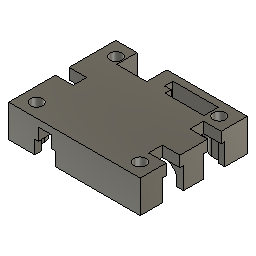
cover servo module (Autodesk Fusion 360 design; units mm, degrees)
Autodesk Fusion 360 part; units mm, degrees
note: some values were not read from the file. Set by a fixed rule: which sketch regions a step uses.
sketch "Skizze1" plane through (0, 0, 0) normal (0, 0, 1) x (1, 0, 0)
  line L0 (24.25, -19.75) -> (-24.25, -19.75)
  line L1 (-24.25, -19.75) -> (-24.25, 19.75)
  line L2 (-24.25, 19.75) -> (24.25, 19.75)
  line L3 (24.25, 19.75) -> (24.25, -19.75)
  line L4 (24.25, -19.75) -> (-24.25, 19.75) construction
  line L5 (-24.25, -19.75) -> (24.25, 19.75) construction
  dimension "d1" = 48.5
  dimension "d2" = 39.5
  constraint horizontal L0
  constraint perpendicular L0 L1
  constraint parallel L0 L2
  constraint parallel L1 L3
  constraint coincident L4 origin
  constraint coincident L5 origin
  measures "d1" distance of L1.end L2.end
  measures "d2" distance of L0.end L1.end
extrude "Extrusion1" add sketch "Skizze1" along normal blind 12
sketch "Skizze2" plane through (0, 0, 0) normal (0, 0, -1) x (1, 0, 0)
  line L0 (-24.25, -19.75) -> (24.25, -19.75)
  line L1 (24.25, -19.75) -> (24.25, 19.75)
  line L2 (24.25, 19.75) -> (-24.25, 19.75)
  line L3 (-24.25, 19.75) -> (-24.25, -19.75)
  line L4 (-21.75, 17.25) -> (21.75, 17.25)
  line L5 (21.75, 17.25) -> (21.75, -17.25)
  line L6 (21.75, -17.25) -> (-21.75, -17.25)
  line L7 (-21.75, -17.25) -> (-21.75, 17.25)
  line L8 (-21.75, 17.25) -> (21.75, -17.25) construction
  line L9 (21.75, 17.25) -> (-21.75, -17.25) construction
  dimension "d5" = 43.5
  dimension "d6" = 34.5
  constraint horizontal L4
  constraint perpendicular L4 L5
  constraint parallel L4 L6
  constraint parallel L5 L7
  constraint coincident L8 origin
  constraint coincident L9 origin
  measures "d5" distance of L5.end L6.end
  measures "d6" distance of L4.end L5.end
extrude "Extrusion2" cut sketch "Skizze2" against normal up to surface (10.5 mm away) contours L4 L5 L6 L7
sketch "Skizze4" plane through (0, 0, 10.5) normal (0, 0, -1) x (1, 0, 0)
  line L0 (21.75, -17.25) -> (21.75, 17.25)
  line L1 (21.75, 17.25) -> (-21.75, 17.25)
  line L2 (-21.75, 17.25) -> (-21.75, -17.25)
  line L3 (-21.75, -17.25) -> (21.75, -17.25)
  line L4 (-21.75, -17.25) -> (-16.05, -17.25)
  line L5 (-16.05, -17.25) -> (-16.05, -14.605)
  line L6 (-19.05, -11.605) -> (-21.75, -11.605)
  line L7 (-21.75, -11.605) -> (-21.75, -17.25)
  line L8 (-21.75, 17.25) -> (-16.05, 17.25)
  line L9 (-16.05, 17.25) -> (-16.05, 14.605)
  line L10 (-19.05, 11.605) -> (-21.75, 11.605)
  line L11 (-21.75, 11.605) -> (-21.75, 17.25)
  line L12 (21.75, 17.25) -> (16.05, 17.25)
  line L13 (16.05, 17.25) -> (16.05, 14.605)
  line L14 (19.05, 11.605) -> (21.75, 11.605)
  line L15 (21.75, 11.605) -> (21.75, 17.25)
  line L16 (21.75, -17.25) -> (16.05, -17.25)
  line L17 (16.05, -17.25) -> (16.05, -14.605)
  line L18 (19.05, -11.605) -> (21.75, -11.605)
  line L19 (21.75, -11.605) -> (21.75, -17.25)
  arc A0 (-19.05, 11.605) -> (-16.05, 14.605) centre (-19.05, 14.605) ccw
  arc A1 (16.05, 14.605) -> (19.05, 11.605) centre (19.05, 14.605) ccw
  arc A2 (19.05, -11.605) -> (16.05, -14.605) centre (19.05, -14.605) ccw
  arc A3 (-16.05, -14.605) -> (-19.05, -11.605) centre (-19.05, -14.605) ccw
  dimension "d9" = 3
  dimension "d10" = 29.21
  dimension "d11" = 38.1
  constraint horizontal L4
  constraint vertical L5
  constraint horizontal L6
  constraint vertical L7
  constraint coincident L2.end L3.start
  constraint horizontal L8
  constraint vertical L9
  constraint horizontal L10
  constraint vertical L11
  constraint coincident L1.end L2.start
  constraint horizontal L12
  constraint vertical L13
  constraint horizontal L14
  constraint vertical L15
  constraint coincident L0.end L1.start
  constraint horizontal L16
  constraint vertical L17
  constraint horizontal L18
  constraint vertical L19
  constraint coincident L0.start L3.end
  constraint tangent L9 A0
  constraint tangent L10 A0
  constraint tangent L13 A1
  constraint tangent L14 A1
  constraint equal A0 A1
  constraint tangent L17 A2
  constraint tangent L18 A2
  constraint equal A0 A2
  constraint tangent L5 A3
  constraint tangent L6 A3
  constraint equal A0 A3
  constraint collinear L6 L18
  constraint collinear L10 L14
  constraint collinear L5 L9
  constraint collinear L13 L17
  constraint equal L10 L14
  constraint equal L5 L9
  measures "d9" radius of A0
  measures "d10" distance of A0.centre A3.centre
  measures "d11" distance of A2.centre A3.centre
extrude "Extrusion3" add sketch "Skizze4" along normal up to surface (9.75 mm away) contours L0 L3 L16 L17 L18 L19 A2 | L0 L1 L12 L13 L14 L15 A1 | L2 L3 L4 L5 L6 L7 A3 | L1 L2 L8 L9 L10 L11 A0
hole "Bohrung1" at (-19.05, -14.605, 12) direction (0, 0, -1) diameter 2.5 end through all counterbore diameter 4.5 counterbore depth 6
mirror "Spiegeln1" about plane through (0, 0, 0) normal (1, 0, 0) of "Bohrung1"
mirror "Spiegeln2" about plane through (0, 0, 0) normal (0, 1, 0) of "Bohrung1", "Spiegeln1"
sketch "Skizze5" plane through (24.25, 0, 0) normal (1, 0, 0) x (0, 1, 0)
  line L0 (-19.75, 12) -> (-19.75, 0)
  line L1 (-19.75, 0) -> (19.75, 0)
  line L2 (19.75, 0) -> (19.75, 12)
  line L3 (-3.77, 0) -> (-11.47, 0)
  line L4 (-11.47, 0) -> (-11.47, 8)
  line L5 (-11.47, 8) -> (-3.77, 8)
  line L6 (-3.77, 8) -> (-3.77, 0)
  line L7 (19.75, 12) -> (-19.75, 12)
  point P0 (-7.62, 0)
  dimension "d22" = 7.7
  dimension "d23" = 7.62
  dimension "d24" = 8
  constraint horizontal L3
  constraint vertical L4
  constraint horizontal L5
  constraint vertical L6
  constraint coincident L1 L3.start
  constraint midpoint L3 P0
  measures "d22" distance of L3.start L3.end
  measures "d23" distance of origin P0
  measures "d24" distance of L3.end L4.end
extrude "Extrusion4" cut sketch "Skizze5" against normal up to surface (2.5 mm away) contours L1 L3 L4 L5 L6
sketch "Skizze7" plane through (0, 0, 10.5) normal (0, 0, -1) x (1, 0, 0)
  line L0 (21.75, 11.605) -> (19.05, 11.605)
  arc A0 (16.05, 14.605) -> (19.05, 11.605) centre (19.05, 14.605) ccw
  line L1 (16.05, 14.605) -> (16.05, 17.25)
  line L2 (16.05, 17.25) -> (-16.05, 17.25)
  line L3 (-16.05, 17.25) -> (-16.05, 14.605)
  arc A1 (-19.05, 11.605) -> (-16.05, 14.605) centre (-19.05, 14.605) ccw
  line L4 (-19.05, 11.605) -> (-21.75, 11.605)
  line L5 (-21.75, 11.605) -> (-21.75, -11.605)
  line L6 (-21.75, -11.605) -> (-19.05, -11.605)
  arc A2 (-16.05, -14.605) -> (-19.05, -11.605) centre (-19.05, -14.605) ccw
  line L7 (-16.05, -14.605) -> (-16.05, -17.25)
  line L8 (-16.05, -17.25) -> (16.05, -17.25)
  line L9 (16.05, -17.25) -> (16.05, -14.605)
  arc A3 (19.05, -11.605) -> (16.05, -14.605) centre (19.05, -14.605) ccw
  line L10 (19.05, -11.605) -> (21.75, -11.605)
  line L11 (21.75, -11.605) -> (21.75, 11.605)
  line L12 (16.05, 14.605) -> (16.05, -14.605)
  constraint vertical L12
  constraint collinear L1 L12
  constraint coincident A0.start L1.start
  constraint coincident L9.end A3.end
extrude "Extrusion6" add sketch "Skizze7" along normal up to surface (2.5 mm away) contours L0 A0 A3 L10 L11 L12
sketch "Skizze6" plane through (24.25, 0, 0) normal (1, 0, 0) x (0, 1, 0)
  line L0 (-11.47, 0) -> (-11.47, 8)
  line L1 (-11.47, 8) -> (-3.77, 8)
  line L2 (-3.77, 8) -> (-3.77, 0)
  line L3 (-3.77, 0) -> (19.75, 0)
  line L4 (19.75, 0) -> (19.75, 12)
  line L5 (-19.75, 12) -> (-19.75, 0)
  line L6 (-19.75, 0) -> (-11.47, 0)
  line L7 (-10.12, 8) -> (-5.12, 8)
  line L8 (-5.12, 8) -> (-5.12, 12)
  line L9 (-5.12, 12) -> (-10.12, 12)
  line L10 (-10.12, 12) -> (-10.12, 8)
  line L11 (19.75, 12) -> (-19.75, 12)
  dimension "d27" = 5
  constraint horizontal L7
  constraint vertical L8
  constraint horizontal L9
  constraint vertical L10
  constraint coincident L1 L7.start
  constraint midpoint L1 L7
  constraint collinear L9 L11
  measures "d27" distance of L8.end L9.end
extrude "Extrusion5" cut sketch "Skizze6" against normal blind 6.5 contours L1 L7 L8 L9 L10 L11
mirror "Spiegeln5" about plane through (0, 0, 0) normal (0, 1, 0) of "Extrusion4", "Extrusion5"
sketch "Skizze8" plane through (-24.25, 0, 0) normal (-1, 0, 0) x (0, -1, 0)
  line L0 (-19.75, 12) -> (-19.75, 0)
  line L1 (-19.75, 0) -> (19.75, 0)
  line L2 (19.75, 0) -> (19.75, 12)
  line L3 (-9.75, 0) -> (9.75, 0)
  line L4 (9.75, 0) -> (9.75, 8)
  line L5 (9.75, 8) -> (-9.75, 8)
  line L6 (-9.75, 8) -> (-9.75, 0)
  line L7 (19.75, 12) -> (-19.75, 12)
  line L8 (-11.47, 8, -48.5) -> (-11.47, 0, -48.5)
  dimension "d35" = 19.5
  constraint horizontal L3
  constraint vertical L4
  constraint horizontal L5
  constraint vertical L6
  constraint coincident L1 L3.start
  constraint midpoint L1 L3
  measures "d35" distance of L4.end L5.end
extrude "Extrusion7" cut sketch "Skizze8" against normal up to surface (2.5 mm away) contours L1 L3 L4 L5 L6
chamfer "Fase2" distance 4 angle 45 1 edges at (21.75, 0, 8)
fillet "Abrundung1" radius 3 2 edges at (21.75, 0, 4) (17.75, 0, 8)
sketch "Skizze16" plane through (0, 0, 10.5) normal (0, 0, -1) x (1, 0, 0)
  line L0 (16.05, -17.25) -> (16.05, 17.25)
  line L1 (16.05, 17.25) -> (-16.05, 17.25)
  line L2 (-16.05, 17.25) -> (-16.05, 14.605)
  arc A0 (-19.05, 11.605) -> (-16.05, 14.605) centre (-19.05, 14.605) ccw
  line L3 (-19.05, 11.605) -> (-21.75, 11.605)
  line L4 (-21.75, 11.605) -> (-21.75, -11.605)
  line L5 (-21.75, -11.605) -> (-19.05, -11.605)
  arc A1 (-16.05, -14.605) -> (-19.05, -11.605) centre (-19.05, -14.605) ccw
  line L6 (-16.05, -14.605) -> (-16.05, -17.25)
  line L7 (-16.05, -17.25) -> (16.05, -17.25)
  line L8 (-16.05, -14.605) -> (-16.05, 14.605)
  constraint coincident A1.start L6.start
  constraint coincident L2.end A0.end
extrude "Extrusion11" add sketch "Skizze16" along normal up to surface (2.5 mm away) contours A0 L3 L4 L5 A1 L8
sketch "Skizze15" plane through (-24.25, 0, 0) normal (-1, 0, 0) x (0, -1, 0)
  line L0 (9.75, 8) -> (9.75, 0)
  line L1 (9.75, 0) -> (19.75, 0)
  line L2 (19.75, 0) -> (19.75, 12)
  line L3 (19.75, 12) -> (-19.75, 12)
  line L4 (-19.75, 12) -> (-19.75, 0)
  line L5 (-19.75, 0) -> (-9.75, 0)
  line L6 (-9.75, 0) -> (-9.75, 8)
  line L7 (-9.75, 8) -> (9.75, 8)
  line L8 (-2.5, 12) -> (2.5, 12)
  line L9 (2.5, 12) -> (2.5, 8)
  line L10 (2.5, 8) -> (-2.5, 8)
  line L11 (-2.5, 8) -> (-2.5, 12)
  dimension "d52" = 5
  constraint horizontal L8
  constraint vertical L9
  constraint horizontal L10
  constraint vertical L11
  constraint coincident L7 L9.end
  constraint coincident L3 L8.start
  constraint midpoint L3 L8
  measures "d52" distance of L8.start L8.end
extrude "Extrusion10" cut sketch "Skizze15" against normal blind 6.5 contours L3 L7 L8 L9 L10 L11
sketch "Skizze17" plane through (0, 0, 10.5) normal (0, 0, -1) x (1, 0, 0)
  line L0 (-16.05, 17.25) -> (-16.05, -17.25)
  line L1 (-16.05, -17.25) -> (16.05, -17.25)
  line L2 (16.05, -17.25) -> (16.05, 17.25)
  line L3 (16.05, 17.25) -> (-16.05, 17.25)
  line L4 (1.73, -17.25) -> (16.05, -17.25)
  line L5 (16.05, -17.25) -> (16.05, -11.96)
  line L6 (16.05, -11.96) -> (1.73, -11.96)
  line L7 (1.73, -11.96) -> (1.73, -17.25)
  line L8 (1.73, -17.25) -> (16.05, -11.96) construction
  line L9 (16.05, -17.25) -> (1.73, -11.96) construction
  line L10 (1.73, -17.25) -> (-0.67, -17.25)
  line L11 (-0.67, -17.25) -> (-0.67, -14.205)
  line L12 (-0.67, -14.205) -> (1.73, -14.205)
  line L13 (1.73, -14.205) -> (1.73, -17.25)
  circle A0 centre (19.05, -14.605) radius 1.25
  line L14 (8.89, -14.605) -> (13.97, -14.605) construction
  line L15 (13.97, -14.605) -> (19.05, -14.605) construction
  point P0 (8.89, -14.605)
  point P1 (1.73, -14.605)
  dimension "d65" = 0.4
  dimension "d66" = 2.4
  dimension "d68" = 5.08
  dimension "d71" = 5.08
  constraint horizontal L4
  constraint perpendicular L4 L5
  constraint parallel L4 L6
  constraint coincident L8 P0
  constraint coincident L9 P0
  constraint horizontal L10
  constraint vertical L11
  constraint horizontal L12
  constraint vertical L13
  constraint midpoint L7 P1
  constraint coincident L7 L12.end
  constraint coincident P0 L14.start
  constraint coincident A0.centre L15.end
  constraint horizontal L15
  constraint horizontal L14
  constraint coincident L1.end L2.start
  measures "d65" distance of L12 P1
  measures "d66" distance of L11.end L12.end
  measures "d68" distance of P0 L14.end
  measures "d71" horizontal distance of L14.end A0.centre
extrude "Extrusion12" cut sketch "Skizze17" against normal through all contours L1 L7 L10 L11 L12 L13 | L1 L2 L4 L5 L6 L7 L13
sketch "Skizze18" plane through (0, 0, 10.5) normal (0, 0, -1) x (1, 0, 0)
  line L0 (1.73, -11.96) -> (16.05, -11.96)
  line L1 (16.05, -11.96) -> (16.05, 17.25)
  line L2 (16.05, 17.25) -> (-16.05, 17.25)
  line L3 (-16.05, 17.25) -> (-16.05, -17.25)
  line L4 (-16.05, -17.25) -> (-0.67, -17.25)
  line L5 (-0.67, -17.25) -> (-0.67, -14.205)
  line L6 (-0.67, -14.205) -> (1.73, -14.205)
  line L7 (1.73, -14.205) -> (1.73, -11.96)
  line L8 (14.05, -11.96) -> (14.05, -9.96)
  line L9 (14.05, -9.96) -> (-2.67, -9.96)
  line L10 (-2.67, -9.96) -> (-2.67, -17.25)
  dimension "d72" = 2
  dimension "d73" = 2
  dimension "d74" = 2
  constraint coincident L0 L8.start
  constraint perpendicular L0 L8
  constraint perpendicular L8 L9
  constraint coincident L4 L10.end
  constraint perpendicular L4 L10
  measures "d72" distance of L5 L10
  measures "d73" distance of L8.start L8.end
  measures "d74" distance of L1 L8
extrude "Extrusion13" add sketch "Skizze18" along normal blind 6 contours L0 L4 L5 L6 L7 L8 L9 L10
sketch "Skizze19" plane through (0, -19.75, 0) normal (0, -1, 0) x (1, 0, 0)
  line L0 (-24.25, 0) -> (24.25, 0)
  line L1 (24.25, 0) -> (24.25, 12)
  line L2 (24.25, 12) -> (-24.25, 12)
  line L3 (-24.25, 12) -> (-24.25, 0)
  line L4 (-14.65, 0) -> (-6.95, 0)
  line L5 (-6.95, 0) -> (-6.95, 5)
  line L6 (-6.95, 5) -> (-14.65, 5)
  line L7 (-14.65, 5) -> (-14.65, 0)
  line L8 (-17.8, 0.75) -> (-20.3, 0.75)
  line L9 (-19.05, 0.75) -> (-19.05, 0) construction
  point P0 (-10.8, 0)
  dimension "d77" = 7.7
  dimension "d78" = 5
  dimension "d79" = 8.25
  constraint horizontal L4
  constraint vertical L5
  constraint horizontal L6
  constraint vertical L7
  constraint coincident L0 L4.start
  constraint midpoint L4 P0
  constraint midpoint L8 L9.start
  constraint coincident L0 L9.end
  constraint perpendicular L0 L9
  measures "d77" distance of L4.start L4.end
  measures "d78" distance of L4.start L6.end
  measures "d79" distance of P0 L9
extrude "Extrusion14" cut sketch "Skizze19" against normal up to surface (2.5 mm away) contours L0 L4 L5 L6 L7
sketch "Skizze20" plane through (0, 0, 10.5) normal (0, 0, -1) x (1, 0, 0)
  line L0 (14.05, -9.96) -> (14.05, -11.96)
  line L1 (14.05, -11.96) -> (16.05, -11.96)
  line L2 (16.05, -11.96) -> (16.05, 17.25)
  line L3 (16.05, 17.25) -> (-16.05, 17.25)
  line L4 (-16.05, 17.25) -> (-16.05, -17.25)
  line L5 (-16.05, -17.25) -> (-2.67, -17.25)
  line L6 (-2.67, -17.25) -> (-2.67, -9.96)
  line L7 (-2.67, -9.96) -> (14.05, -9.96)
  line L8 (-19.05, 11.605) -> (-5.8, 11.605)
  line L9 (-5.8, 11.605) -> (-5.8, 17.25)
  arc A0 (-19.05, 11.605) -> (-16.05, 14.605) centre (-19.05, 14.605) ccw
  line L10 (-16.05, 14.605) -> (-16.05, 17.25)
  circle A1 centre (-19.05, 14.605) radius 3
  point P0 (-6.95, 17.25)
  point P1 (-19.05, 11.605)
  dimension "d82" = 1.15
  constraint coincident L3 L9.end
  constraint perpendicular L3 L9
  constraint coincident P1 L8.start
  constraint perpendicular L8 L9
  constraint coincident A0.end L10.start
  constraint coincident L3.end L4.start
  constraint concentric A0 A1
  constraint coincident P1 A1
  measures "d82" distance of L9 P0
extrude "Extrusion15" add sketch "Skizze20" along normal up to surface (5.5 mm away) contours L3 L4 L8 L9 L10 | L4 L8 A0 A1
sketch "Skizze21" plane through (0, 0, 5) normal (0, 0, -1) x (1, 0, 0)
  line L0 (-6.95, 17.25) -> (-6.95, 19.75)
  line L1 (-6.95, 19.75) -> (-14.65, 19.75)
  line L2 (-14.65, 19.75) -> (-14.65, 17.25)
  line L3 (-14.65, 17.25) -> (-16.05, 17.25)
  line L4 (-16.05, 17.25) -> (-16.05, 14.605)
  arc A0 (-19.05, 11.605) -> (-16.05, 14.605) centre (-19.05, 14.605) ccw
  line L5 (-19.05, 11.605) -> (-5.8, 11.605)
  line L6 (-5.8, 11.605) -> (-5.8, 17.25)
  line L7 (-5.8, 17.25) -> (-6.95, 17.25)
  line L8 (-13.3, 19.75) -> (-8.3, 19.75)
  line L9 (-8.3, 19.75) -> (-8.3, 13.25)
  line L10 (-8.3, 13.25) -> (-13.3, 13.25)
  line L11 (-13.3, 13.25) -> (-13.3, 19.75)
  dimension "d85" = 5
  dimension "d86" = 6.5
  constraint horizontal L8
  constraint vertical L9
  constraint horizontal L10
  constraint vertical L11
  constraint coincident L1 L8.start
  constraint midpoint L1 L8
  measures "d85" distance of L8.start L8.end
  measures "d86" distance of L8.start L10.end
extrude "Extrusion16" cut sketch "Skizze21" against normal blind 4.5 contours L1 L8 L9 L10 L11
sketch "Skizze22" plane through (0, 19.75, 0) normal (0, 1, 0) x (-1, 0, 0)
  line L0 (-24.25, 0) -> (24.25, 0)
  line L1 (24.25, 0) -> (24.25, 12)
  line L2 (24.25, 12) -> (-24.25, 12)
  line L3 (-24.25, 12) -> (-24.25, 0)
  line L4 (16.4, 0) -> (5.4, 0)
  line L5 (5.4, 0) -> (5.4, 9)
  line L6 (5.4, 9) -> (16.4, 9)
  line L7 (16.4, 9) -> (16.4, 0)
  line L8 (20.3, 0.75) -> (17.8, 0.75)
  line L9 (19.05, 0.75) -> (19.05, 0) construction
  point P0 (10.9, 0)
  dimension "d89" = 11
  dimension "d90" = 9
  dimension "d91" = 8.15
  constraint horizontal L4
  constraint vertical L5
  constraint horizontal L6
  constraint vertical L7
  constraint coincident L0 L4.start
  constraint midpoint L8 L9.start
  constraint coincident L0 L9.end
  constraint perpendicular L0 L9
  constraint midpoint L4 P0
  measures "d89" distance of L4.start L4.end
  measures "d90" distance of L4.start L6.end
  measures "d91" distance of L9 P0
extrude "Extrusion17" cut sketch "Skizze22" against normal blind 10 contours L0 L4 L5 L6 L7
sketch "Skizze23" plane through (0, 0, 9) normal (0, 0, -1) x (1, 0, 0)
  line L0 (-5.4, -17.25) -> (-16.05, -17.25)
  line L1 (-16.05, -17.25) -> (-16.05, -9.75)
  line L2 (-16.05, -9.75) -> (-16.4, -9.75)
  line L3 (-16.4, -9.75) -> (-16.4, -19.75)
  line L4 (-16.4, -19.75) -> (-5.4, -19.75)
  line L5 (-5.4, -19.75) -> (-5.4, -17.25)
  line L6 (-16.4, -19.75) -> (-5.4, -19.75)
  line L7 (-5.4, -19.75) -> (-5.4, -12.25)
  line L8 (-5.4, -12.25) -> (-16.4, -12.25)
  line L9 (-16.4, -12.25) -> (-16.4, -19.75)
  dimension "d95" = 7.5
  constraint horizontal L6
  constraint vertical L7
  constraint horizontal L8
  constraint vertical L9
  constraint coincident L3.end L4.start
  constraint coincident L4.end L5.start
  measures "d95" distance of L7.end L4.end
extrude "Extrusion18" cut sketch "Skizze23" against normal through all contours L0 L1 L3 L4 L5 L6 L7 L8 L9 | L0 L1 L7 L8
equation "d23 = ( 15.24 / 2 ) * 1 mm"
equation "d73 = d72"
named bodies: "Motor Deckel"
